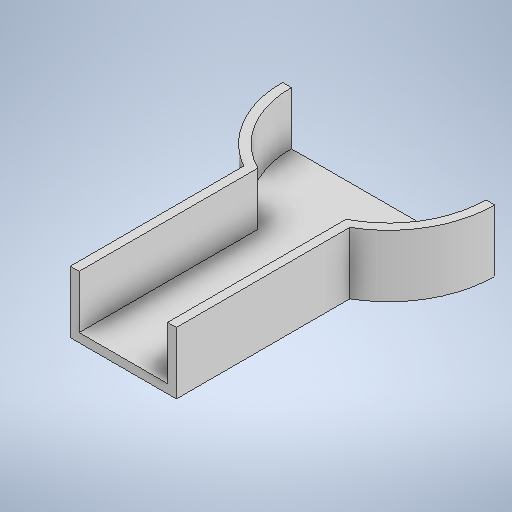
# Autodesk Inventor part: select end track
Saved by Autodesk Inventor 2025.3 (Build 293356000, 356)
## iProperties
Created: 2026-04-19
Part Number: select end track
Material: Generic
Document SubType Name: Modeling
Designer: kamal
Density: 1 g/cm^3
Appearance: Default
Author: kamal
Autodesk Inventor part; units mm, degrees
ref_plane "YZ Plane" through (0, 0, 0) normal (1, 0, 0) x (0, 1, 0)
ref_plane "XZ Plane" through (0, 0, 0) normal (0, 1, 0) x (-1, 0, 0)
ref_plane "XY Plane" through (0, 0, 0) normal (0, 0, 1) x (1, 0, 0)
sketch "Sketch1" plane through (0, 0, 0) normal (0, 0, 1) x (1, 0, 0)
  line L0 (-60, -17.5) -> (0, -17.5)
  line L1 (60, -17.5) -> (60, 17.5) construction
  line L2 (60, 17.5) -> (55, 17.5) construction
  line L3 (-60, 17.5) -> (-60, -17.5)
  line L4 (-60, -17.5) -> (60, 17.5) construction
  line L5 (60, -17.5) -> (-60, 17.5) construction
  line L6 (-55, -12.5) -> (0, -12.5)
  line L7 (55, -12.5) -> (55, 12.5) construction
  line L8 (55, 12.5) -> (-55, 12.5) construction
  line L9 (-55, 12.5) -> (-55, -12.5)
  line L10 (-55, 12.5) -> (-55, 17.5)
  line L11 (55, 12.5) -> (55, 17.5) construction
  line L12 (-55, 17.5) -> (-60, 17.5)
  line L13 (55, 17.5) -> (-55, 17.5) construction
  line L14 (0, -17.5) -> (0, 17.5)
  line L15 (0, -12.5) -> (55, -12.5) construction
  line L16 (0, -17.5) -> (60, -17.5) construction
  line L17 (0, -12.5) -> (0, -17.5)
  line L18 (0, 17.5) -> (-55, 17.5)
  point P0 (0, 0)
  dimension "d0" = 120
  dimension "d1" = 35
  dimension "d2" = 5
  dimension "d3" = 5
  dimension "d4" = 5
  dimension "d5" = 30
  constraints: 38 end point, 12 perpendicular, 11 parallel, 3 midpoint, 2 horizontal, 1 point on line
  measures "d0" distance of L3.start L1.end
  measures "d1" distance of L1.start L1.end
  measures "d2" distance between parallel lines of L3 L9
  measures "d3" distance between parallel lines of L7 L1
  measures "d4" distance between parallel lines of L8 L12
  measures "d5" distance between parallel lines of L15 L13
revolve "Revolution1" add sketch "Sketch1" angle 180 about axis through (0, -17.5, 0) along (0, 1, 0) contours L3 L12 L10 L9 L6 L14 L0
sketch "Sketch2" plane through (60, -17.5, 0) normal (0, 0, -1) x (-1, 0, 0)
  line L0 (0, 35) -> (0, 0) projected
  line L1 (0, 0) -> (60, 0) construction
  line L2 (120, 0) -> (0, 0) projected
  line L3 (60, 0) -> (60, 35) construction
  line L4 (60, 0) -> (60, 5) construction
  line L5 (60, 5) -> (35, 5)
  line L6 (35, 5) -> (35, 35)
  line L7 (35, 35) -> (30, 35)
  line L8 (30, 35) -> (30, 0)
  line L9 (60, 5) -> (85, 5)
  line L10 (85, 5) -> (85, 35)
  line L11 (85, 35) -> (90, 35)
  line L12 (90, 35) -> (90, 0)
  point P0 (60, 17.5)
  dimension "d7" = 60
  dimension "d8" = 35
  dimension "d9" = 5
  dimension "d10" = 25
  dimension "d11" = 30
  dimension "d12" = 5
  constraints: 22 end point, 4 perpendicular, 4 symmetric about line, 2 point on line, 1 midpoint, 1 parallel
  measures "d7" distance of L0.end L1.end
  measures "d8" distance of L1.end L3.end
  measures "d9" distance of L1.end L4.end
  measures "d10" distance of L4.end L5.end
  measures "d11" distance of L5.end L6.end
  measures "d12" distance of L6.end L7.end
extrude "Extrusion1" add sketch "Sketch2" against normal blind 150
sketch "Sketch3" plane through (60, -17.5, 0) normal (0, 0, -1) x (-1, 0, 0)
  line L0 (35, 35) -> (35, 5) projected
  line L1 (85, 5) -> (35, 5) projected
  line L2 (85, 5) -> (85, 35) projected
  line L3 (85, 35) -> (35, 35) projected
  point P0 (60, 17.5)
extrude "Extrusion2" cut sketch "Sketch3" against normal through all
revolve "Revolution2" cut sketch "Sketch1" angle 360 about axis through (0, -17.5, 0) along (0, 1, 0) contours L6 L9 L10 L18 L14
body "Solid1"
